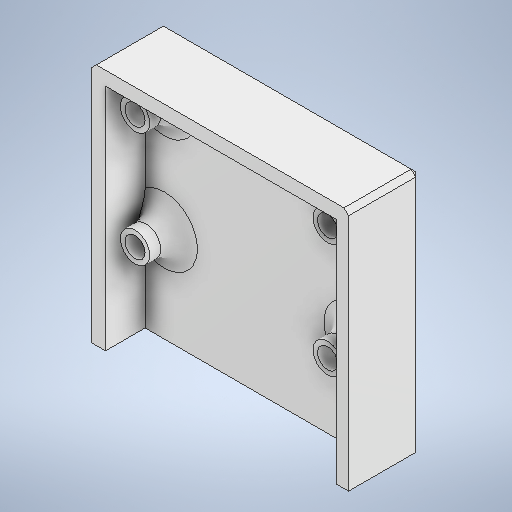
# Autodesk Inventor part: Base
Saved by Autodesk Inventor 2025.2 (Build 292293000, 293)
## iProperties
Created: 2025-04-01
Part Number: Base
Material: PC/ABS Plastic
Document SubType Name: Modeling
Designer: franc
Density: 1.1 g/cm^3
Appearance: Smooth - White
Author: franc
Autodesk Inventor part; units mm, degrees
ref_plane "YZ Plane" through (0, 0, 0) normal (1, 0, 0) x (0, 1, 0)
ref_plane "XZ Plane" through (0, 0, 0) normal (0, 1, 0) x (-1, 0, 0)
ref_plane "XY Plane" through (0, 0, 0) normal (0, 0, 1) x (1, 0, 0)
sketch "Sketch1" plane through (0, 0, 0) normal (0, 0, 1) x (1, 0, 0)
  line L0 (0, 0) -> (-25.2, 0)
  line L1 (-25.2, 0) -> (-25.2, 25)
  line L2 (-25.2, 25) -> (0, 25)
  line L3 (0, 25) -> (0, 0)
  circle A0 centre (-23.1, 22.8) radius 1.1
  circle A1 centre (-2.1, 22.8) radius 1.1
  circle A2 centre (-23.1, 10.3) radius 1.1
  circle A3 centre (-2.1, 10.3) radius 1.1
  dimension "d2" = 2.2
  dimension "d5" = 2.2
  dimension "d7" = 12.5
  dimension "d8" = 2.2
  dimension "d9" = 2.2
  dimension "d14" = 12.5
  dimension "d29" = 25.2
  dimension "d31" = 2.1
  dimension "d32" = 2.1
  constraints: 8 end point, 4 centre point, 2 parallel, 1 coincident, 1 horizontal, 1 perpendicular
  measures "d2" diameter of A0
  measures "d5" diameter of A1
  measures "d7" distance of point (-23.1, 10.3) A0.centre
  measures "d8" diameter of A2
  measures "d9" diameter of A3
  measures "d14" distance of A3.centre A1.centre
  measures "d29" distance between parallel lines of L3 L1
  measures "d31" distance from line of L3 A1.centre
  measures "d32" distance from line of A0.centre L1
extrude "Base" add sketch "Sketch1" along normal blind 3.5
sketch "Sketch2" plane through (0, 0, 3.5) normal (0, 0, 1) x (1, 0, 0)
  line L0 (-25.2, 25) -> (-25.2, 0) projected
  line L1 (-25.2, 0) -> (-26.7, 0)
  line L2 (-26.7, 0) -> (-26.7, 26.5)
  line L3 (-26.7, 26.5) -> (1.3, 26.5)
  line L4 (1.3, 26.5) -> (1.3, 0)
  line L5 (1.3, 0) -> (0, 0)
  line L6 (0, 25) -> (-25.2, 25) projected
  line L7 (0, 0) -> (0, 25) projected
  dimension "d15" = 1.5
  dimension "d16" = 26.5
  dimension "d17" = 28
  constraints: 10 end point, 4 perpendicular, 1 horizontal, 1 point on line
  measures "d15" distance of L0.end L1.end
  measures "d16" distance of L1.end L2.end
  measures "d17" distance of L2.end L3.end
extrude "Walls" add sketch "Sketch2" along normal blind 4.32 and the other way blind 3.5
sketch "Sketch3" plane through (0, 0, 3.5) normal (0, 0, 1) x (1, 0, 0)
  circle A0 centre (-23.1, 10.3) radius 1.1 projected
  circle A1 centre (-23.1, 10.3) radius 1.6
  circle A2 centre (-2.1, 10.3) radius 1.1 projected
  circle A3 centre (-2.1, 10.3) radius 1.6
  circle A4 centre (-23.1, 22.8) radius 1.1 projected
  circle A5 centre (-23.1, 22.8) radius 1.6
  circle A6 centre (-2.1, 22.8) radius 1.1 projected
  circle A7 centre (-2.1, 22.8) radius 1.6
  point P0 (0, 0)
  dimension "d22" = 3.2
  dimension "d23" = 3.2
  dimension "d24" = 3.2
  dimension "d25" = 3.2
  constraints: 4 centre point, 4 coincident
  measures "d22" diameter of A1
  measures "d23" diameter of A3
  measures "d24" diameter of A5
  measures "d25" diameter of A7
extrude "Spacers" add sketch "Sketch3" along normal blind 3.2
fillet "Fillet1" radius 2 4 edges at (-24.7, 22.8, 3.5) (-24.7, 10.3, 3.5) (-3.7, 10.3, 3.5) (-3.7, 22.8, 3.5)
chamfer "Chamfer1" distance 0.5 angle 45 5 edges at (-26.7, 26.5, 3.91) (-12.7, 26.5, 0) (1.3, 26.5, 3.91) (1.3, 13.25, 0) (-26.7, 13.25, 0)
body "Solid1"
